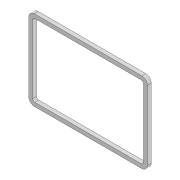
# Autodesk Inventor part: O-Ring Dash 034 Square
Saved by Autodesk Inventor 2020 (Build 240168000, 168)
## iProperties
Created: 2020-04-26
Part Number: O-Ring Dash 034 Square
Material: Generic
Document SubType Name: Modeling
Designer: John K
Density: 1 g/cm^3
Appearance: Default
Author: John K
Autodesk Inventor part; units mm, degrees
ref_plane "YZ Plane" through (0, 0, 0) normal (1, 0, 0) x (0, 1, 0)
ref_plane "XZ Plane" through (0, 0, 0) normal (0, 1, 0) x (-1, 0, 0)
ref_plane "XY Plane" through (0, 0, 0) normal (0, 0, 1) x (1, 0, 0)
sketch "Sketch1" plane through (0, 0, 0) normal (0, 0, 1) x (1, 0, 0)
  line L0 (25.4, -16.637) -> (-25.4, -16.637)
  line L1 (-25.4, -16.637) -> (-25.4, 16.637)
  line L2 (-25.4, 16.637) -> (25.4, 16.637)
  line L3 (25.4, 16.637) -> (25.4, -16.637)
  line L4 (25.4, -16.637) -> (-25.4, 16.637) construction
  line L5 (-25.4, -16.637) -> (25.4, 16.637) construction
  line L6 (27.178, 18.415) -> (-27.178, 18.415)
  line L7 (-27.178, 18.415) -> (-27.178, -18.415)
  line L8 (-27.178, -18.415) -> (27.178, -18.415)
  line L9 (27.178, -18.415) -> (27.178, 18.415)
  point P0 (0, 0)
  dimension "d0" = 50.8
  dimension "d1" = 33.274
  dimension "d2" = 1.778
  constraints: 20 end point, 4 parallel, 2 midpoint, 2 perpendicular, 1 horizontal, 3 other
  measures "d0" distance of L1.end L2.end
  measures "d1" distance of L0.end L1.end
  measures "d2" distance between parallel lines of L2 L6
extrude "Extrusion1" add sketch "Sketch1" along normal mid plane 1.778
fillet "Fillet1" radius 0.9652 4 edges at (25.4, 16.637, 0) (25.4, -16.637, 0) (-25.4, -16.637, 0) (-25.4, 16.637, 0)
fillet "Fillet1" radius 2.54 4 edges at (27.178, -18.415, 0) (27.178, 18.415, 0) (-27.178, 18.415, 0) (-27.178, -18.415, 0)
body "Solid1"
